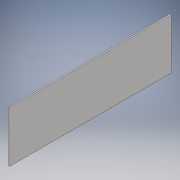
# Autodesk Inventor part: The Robot
Saved by Autodesk Inventor 2017 (Build 210142000, 142)
## iProperties
Created: 2017-06-10
Part Number: The Robot
Material: Generic
Document SubType Name: Modeling
Designer: Matthew
Density: 1 g/cm^3
Appearance: Default
Author: Matthew
Autodesk Inventor part; units mm, degrees
ref_plane "YZ Plane" through (0, 0, 0) normal (1, 0, 0) x (0, 1, 0)
ref_plane "XZ Plane" through (0, 0, 0) normal (0, 1, 0) x (-1, 0, 0)
ref_plane "XY Plane" through (0, 0, 0) normal (0, 0, 1) x (1, 0, 0)
sketch "Sketch1" plane through (0, 0, 0) normal (1, 0, 0) x (0, 1, 0)
  line L0 (5.37, 31.8697) -> (-121.63, 31.8697)
  line L1 (-121.63, 31.8697) -> (-121.63, -374.5303)
  line L2 (-121.63, -374.5303) -> (5.37, -374.5303)
  line L3 (5.37, -374.5303) -> (5.37, 31.8697)
  point P0 (0, 0)
  dimension "d0" = 127
  dimension "d1" = 406.4
  constraints: 8 end point, 2 parallel, 1 horizontal, 1 perpendicular
  measures "d0" distance of L2.end L1.end
  measures "d1" distance of L1.end L0.end
extrude "Extrusion1" add sketch "Sketch1" along normal blind 3.175
body "Solid1"
